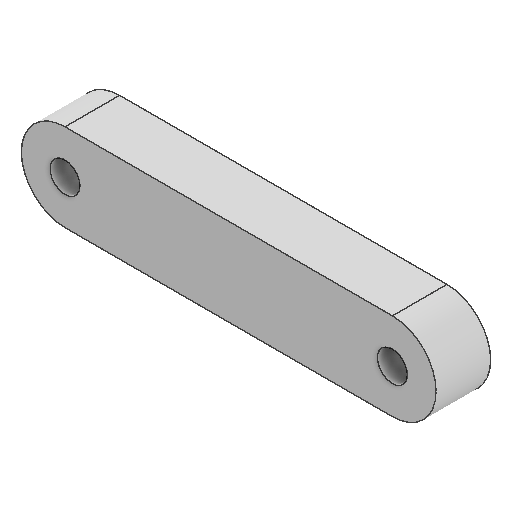
# Autodesk Inventor part: linkB
Saved by Autodesk Inventor 2025 (Build 290162000, 162)
## iProperties
Created: 2025-01-09
Part Number: linkB
Material: Generic
Document SubType Name: Modeling
Designer: derm
Density: 1 g/cm^3
Appearance: Default
Author: derm
Autodesk Inventor part; units mm, degrees
ref_plane "YZ Plane" through (0, 0, 0) normal (1, 0, 0) x (0, 1, 0)
ref_plane "XZ Plane" through (0, 0, 0) normal (0, 1, 0) x (-1, 0, 0)
ref_plane "XY Plane" through (0, 0, 0) normal (0, 0, 1) x (1, 0, 0)
sketch "Sketch1" plane through (0, 0, 0) normal (0, 0, 1) x (1, 0, 0)
  line L0 (0, 0) -> (60, 0) construction
  line L1 (0, -8) -> (60, -8)
  line L2 (60, 8) -> (0, 8)
  arc A0 (0, 8) -> (0, -8) centre (0, 0) ccw
  arc A1 (60, -8) -> (60, 8) centre (60, 0) ccw
  circle A2 centre (0, 0) radius 2.75
  circle A3 centre (60, 0) radius 2.75
  point P0 (30, 0)
  dimension "d0" = 60
  dimension "d1" = 8
  dimension "d2" = 5.5
  constraints: 8 end point, 4 centre point, 4 point on circle, 4 tangent, 2 coincident, 1 equal radius, 1 horizontal, 1 midpoint, 1 parallel
  measures "d0" distance of L0.start L0.end
  measures "d1" radius of A0
  measures "d2" diameter of A3
extrude "Extrusion1" add sketch "Sketch1" along normal blind 10
body "Solid1"
